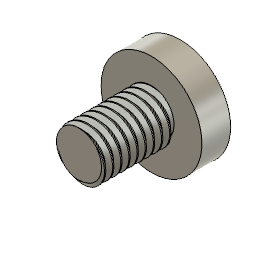
Assembly (Autodesk Fusion 360 archive; units mm, degrees)
design "M5 Screw"
part number: 2025-09-18-13-38-02-357
Autodesk Fusion 360 part; units mm, degrees
sketch "Sketch1" plane through (0, 0, 0) normal (0, 1, 0) x (1, 0, 0)
  line L0 (0, 0) -> (0, 10)
  line L1 (0, 10) -> (4.95, 10)
  line L2 (4.95, 10) -> (4.95, 7.17)
  line L3 (4.95, 7.17) -> (2.45, 7.17)
  line L4 (2.45, 7.17) -> (2.45, 0)
  line L5 (2.45, 0) -> (0, 0)
  dimension "d1" = 10
  dimension "d7" = 4.95
  dimension "d8" = 2.83
  dimension "d10" = 2.45
  constraint coincident L0.start L5.end
  constraint vertical L0
  constraint perpendicular L0 L1
  constraint perpendicular L1 L2
  constraint perpendicular L2 L3
  constraint perpendicular L3 L4
  constraint perpendicular L0 L5
  measures "d1" distance of L0.start L0.end
  measures "d7" distance of L0.end L1.end
  measures "d8" distance of L1.end L2.end
  measures "d10" distance of L0 L4
revolve "Revolve1" add sketch "Sketch1" angle 360 about axis through (0, 0, 0) along (0, 0, -1)
sketch "Sketch2" plane through (0, 0, -10) normal (0, 0, -1) x (-1, 0, 0)
  circle A0 centre (0, 0) radius 4.95
  line L0 (-0.9388, -1.691) -> (0.9951, -1.6585)
  line L1 (0.9951, -1.6585) -> (1.9338, 0.0325)
  line L2 (1.9338, 0.0325) -> (0.9388, 1.691)
  line L3 (0.9388, 1.691) -> (-0.9951, 1.6585)
  line L4 (-0.9951, 1.6585) -> (-1.9338, -0.0325)
  line L5 (-1.9338, -0.0325) -> (-0.9388, -1.691)
  dimension "d12" = 3.35
  constraint coincident A0.centre origin
  measures "d12" distance of L0 L3
extrude "Extrude1" cut sketch "Sketch2" against normal blind 1.2 contours L0 L1 L2 L3 L4 L5
thread "Thread1" "ISO Metric profile 5.0 M5x0.8 M5x0.8 6g" major diameter 4.901 minor diameter 3.9895 pitch 0.8 angle 60 modelled right hand crest width 0.1157 on face at (2.447, 0.1221, -4.78) crest through (2.4505, 0, -7.37)
sketch "Sketch3" plane through (0, 0, -10) normal (0, 0, -1) x (-1, 0, 0)
  line L0 (0.9951, -1.6585) -> (-0.9388, -1.691) construction
  line L1 (-0.9388, -1.691) -> (-1.9338, -0.0325) construction
  line L2 (-1.9338, -0.0325) -> (-0.9951, 1.6585) construction
  line L3 (-0.9951, 1.6585) -> (0.9388, 1.691) construction
  line L4 (0.9388, 1.691) -> (1.9338, 0.0325) construction
  line L5 (1.9338, 0.0325) -> (0.9951, -1.6585) construction
  circle A0 centre (0, 0) radius 4.95
  circle A1 centre (0, 0) radius 1.9341
  constraint coincident A0.centre A1.centre
  constraint coincident L2.end A1
extrude "Extrude2" cut sketch "Sketch3" against normal blind 0.3 draft -45 contours A1
equation "d1 = length"
equation "length = 10 mm"
equation "width = 9.9 mm"
equation "head_height = 2.83 mm"
equation "hole_width = 3.35 mm"
equation "major_diameter = 4.9 mm"
equation "d7 = width / 2"
equation "d8 = head_height"
equation "minor_diameter = 4.1 mm"
equation "d10 = major_diameter / 2"
equation "d12 = hole_width"
equation "thread_pitch = 0.8 mm"
equation "slot_depth = 1.2 mm"
equation "d15 = -slot_depth"
